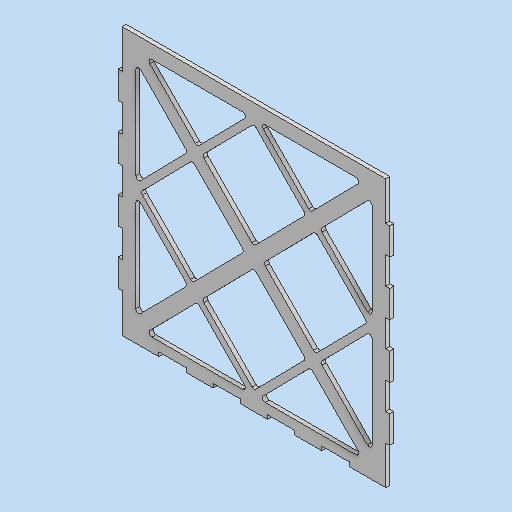
# Autodesk Inventor part: left plate
Saved by Autodesk Inventor 2026 (Build 300175000, 175)
## iProperties
Created: 2026-02-12
Part Number: left plate
Material: Generic
Document SubType Name: Modeling
Designer: mones
Density: 1 g/cm^3
Appearance: Default
Author: mones
Autodesk Inventor part; units mm, degrees
ref_plane "YZ Plane" through (0, 0, 0) normal (1, 0, 0) x (0, 1, 0)
ref_plane "XZ Plane" through (0, 0, 0) normal (0, 1, 0) x (-1, 0, 0)
ref_plane "XY Plane" through (0, 0, 0) normal (0, 0, 1) x (1, 0, 0)
sketch "Sketch1" plane through (0, 0, 0) normal (0, 0, 1) x (1, 0, 0)
  line L0 (-97, 98.5) -> (97, 98.5)
  line L1 (-100, 98.5) -> (100, -98.5) construction
  line L2 (100, 98.5) -> (-100, -98.5) construction
  line L3 (-97, 98.5) -> (-97, 70)
  line L4 (-97, 50) -> (-97, 30)
  line L5 (-97, 10) -> (-97, -10)
  line L6 (-97, -70) -> (-97, -98.5)
  line L7 (-97, 70) -> (-100, 70)
  line L8 (-100, 70) -> (-100, 50)
  line L9 (-100, 30) -> (-100, 10)
  line L10 (-100, -10) -> (-100, -30)
  line L11 (-100, -50) -> (-100, -70)
  line L12 (-100, -70) -> (-97, -70)
  line L13 (-100, -50) -> (-97, -50)
  line L14 (-100, -30) -> (-97, -30)
  line L15 (-100, -10) -> (-97, -10)
  line L16 (-100, 10) -> (-97, 10)
  line L17 (-100, 30) -> (-97, 30)
  line L18 (-100, 50) -> (-97, 50)
  line L19 (97, 98.5) -> (97, 70)
  line L20 (97, 50) -> (97, 30)
  line L21 (97, 10) -> (97, -10)
  line L22 (97, -30) -> (97, -50)
  line L23 (97, -70) -> (97, -98.5)
  line L24 (97, 70) -> (100, 70)
  line L25 (100, 70) -> (100, 50)
  line L26 (100, 30) -> (100, 10)
  line L27 (100, -10) -> (100, -30)
  line L28 (100, -50) -> (100, -70)
  line L29 (100, -70) -> (97, -70)
  line L30 (100, -50) -> (97, -50)
  line L31 (100, -30) -> (97, -30)
  line L32 (100, -10) -> (97, -10)
  line L33 (100, 10) -> (97, 10)
  line L34 (100, 30) -> (97, 30)
  line L35 (100, 50) -> (97, 50)
  line L36 (-100, 50) -> (-100, 70)
  line L37 (-97, 98.5) -> (-97, 70)
  line L38 (-97, 50) -> (-97, 30)
  line L39 (-100, 10) -> (-100, 30)
  line L40 (-97, 10) -> (-97, -10)
  line L41 (-100, -70) -> (-100, -50)
  line L42 (-100, -30) -> (-100, -10)
  line L43 (-97, -30) -> (-97, -50)
  line L44 (-97, -70) -> (-97, -98.5)
  line L45 (100, 50) -> (100, 70)
  line L46 (100, 70) -> (100, 50)
  line L47 (97, 98.5) -> (97, 70)
  line L48 (97, 50) -> (97, 30)
  line L49 (100, 30) -> (100, 10)
  line L50 (100, 10) -> (100, 30)
  line L51 (97, 10) -> (97, -10)
  line L52 (100, -70) -> (100, -50)
  line L53 (100, -30) -> (100, -10)
  line L54 (100, -10) -> (100, -30)
  line L55 (100, -50) -> (100, -70)
  line L56 (97, -30) -> (97, -50)
  line L57 (97, -70) -> (97, -98.5)
  line L58 (-97, -98.5) -> (-70, -98.5)
  line L59 (-50, -98.5) -> (-30, -98.5)
  line L60 (-10, -98.5) -> (10, -98.5)
  line L61 (30, -98.5) -> (50, -98.5)
  line L62 (-97, -98.5) -> (-97, -95.5)
  line L63 (-97, -95.5) -> (97, -95.5) construction
  line L64 (-70, -98.5) -> (-70, -95.5)
  line L65 (-50, -98.5) -> (-50, -95.5)
  line L66 (-30, -98.5) -> (-30, -95.5)
  line L67 (-10, -98.5) -> (-10, -95.5)
  line L68 (10, -98.5) -> (10, -95.5)
  line L69 (30, -98.5) -> (30, -95.5)
  line L70 (50, -98.5) -> (50, -95.5)
  line L71 (70, -98.5) -> (70, -95.5)
  line L72 (97, -98.5) -> (70, -98.5)
  line L73 (50, -95.5) -> (70, -95.5)
  line L74 (50, -98.5) -> (30, -98.5)
  line L75 (10, -95.5) -> (30, -95.5)
  line L76 (10, -98.5) -> (-10, -98.5)
  line L77 (-70, -95.5) -> (-50, -95.5)
  line L78 (-30, -95.5) -> (-10, -95.5)
  line L79 (-30, -98.5) -> (-50, -98.5)
  line L80 (-70, -98.5) -> (-97, -98.5)
  point P0 (0, 0)
  constraints: 160 end point, 58 perpendicular, 28 parallel, 2 midpoint, 2 vertical, 1 horizontal, 1 point on line, 11 other
extrude "Extrusion1" add sketch "Sketch1" along normal blind 3
sketch "Sketch2" plane through (0, 0, 3) normal (0, 0, 1) x (1, 0, 0)
  line L0 (-97, 98.5) -> (-97, 70) projected
  line L1 (-97, 70) -> (-100, 70) projected
  line L2 (-100, 70) -> (-100, 50) projected
  line L3 (-100, 50) -> (-97, 50) projected
  line L4 (-97, 50) -> (-97, 30) projected
  line L5 (-97, 30) -> (-100, 30) projected
  line L6 (-100, 30) -> (-100, 10) projected
  line L7 (-100, 10) -> (-97, 10) projected
  line L8 (-97, 10) -> (-97, -10) projected
  line L9 (-97, -10) -> (-100, -10) projected
  line L10 (-100, -10) -> (-100, -30) projected
  line L11 (-100, -30) -> (-97, -30) projected
  line L12 (-97, -30) -> (-97, -50) projected
  line L13 (-97, -50) -> (-100, -50) projected
  line L14 (-100, -50) -> (-100, -70) projected
  line L15 (-100, -70) -> (-97, -70) projected
  line L16 (-97, -70) -> (-97, -98.5) projected
  line L17 (-97, -98.5) -> (-70, -98.5) projected
  line L18 (-70, -98.5) -> (-70, -95.5) projected
  line L19 (-70, -95.5) -> (-50, -95.5) projected
  line L20 (-50, -95.5) -> (-50, -98.5) projected
  line L21 (-50, -98.5) -> (-30, -98.5) projected
  line L22 (-30, -98.5) -> (-30, -95.5) projected
  line L23 (-30, -95.5) -> (-10, -95.5) projected
  line L24 (-10, -95.5) -> (-10, -98.5) projected
  line L25 (-10, -98.5) -> (10, -98.5) projected
  line L26 (10, -98.5) -> (10, -95.5) projected
  line L27 (10, -95.5) -> (30, -95.5) projected
  line L28 (30, -95.5) -> (30, -98.5) projected
  line L29 (30, -98.5) -> (50, -98.5) projected
  line L30 (50, -98.5) -> (50, -95.5) projected
  line L31 (50, -95.5) -> (70, -95.5) projected
  line L32 (70, -95.5) -> (70, -98.5) projected
  line L33 (70, -98.5) -> (97, -98.5) projected
  line L34 (97, -98.5) -> (97, -70) projected
  line L35 (97, -70) -> (100, -70) projected
  line L36 (100, -70) -> (100, -50) projected
  line L37 (100, -50) -> (97, -50) projected
  line L38 (97, -50) -> (97, -30) projected
  line L39 (97, -30) -> (100, -30) projected
  line L40 (100, -30) -> (100, -10) projected
  line L41 (100, -10) -> (97, -10) projected
  line L42 (97, -10) -> (97, 10) projected
  line L43 (97, 10) -> (100, 10) projected
  line L44 (100, 10) -> (100, 30) projected
  line L45 (100, 30) -> (97, 30) projected
  line L46 (97, 30) -> (97, 50) projected
  line L47 (97, 50) -> (100, 50) projected
  line L48 (100, 50) -> (100, 70) projected
  line L49 (100, 70) -> (97, 70) projected
  line L50 (97, 70) -> (97, 98.5) projected
  line L51 (97, 98.5) -> (-97, 98.5) projected
  line L52 (-97, 98.5) -> (97, 98.5)
  line L53 (97, 98.5) -> (97, -98.5)
  line L54 (97, -98.5) -> (-97, -98.5)
  line L55 (-97, -98.5) -> (-97, 98.5)
  line L56 (-90.5656, -84.9948) -> (90.5656, 84.9948) construction
  line L57 (-90.5656, 84.9948) -> (90.5656, -84.9948) construction
  line L58 (83.4344, -92.0052) -> (-83.4344, 92.0052) construction
  line L59 (1.7528, 86.7169) -> (1.7516, 86.7182)
  line L60 (-88.7828, -1.7526) -> (0, -85.0743) construction
  line L61 (-1.7828, -90.2526) -> (-85.2172, 1.7526) construction
  line L62 (85.2172, 1.7526) -> (1.7828, -90.2526) construction
  line L63 (85.2172, -1.7526) -> (1.7828, 90.2526) construction
  line L64 (-88.7828, 1.7526) -> (1.7828, 86.7474) construction
  line L65 (-1.7828, 90.2526) -> (-85.2172, -1.7526) construction
  line L66 (75.2179, 88.5) -> (8.2764, 88.5)
  line L67 (-8.2764, 88.5) -> (-75.2179, 88.5)
  line L68 (87, -76.4803) -> (87, -8.4535)
  line L69 (87, 8.4535) -> (87, 76.4803)
  line L70 (6.8501, -85.0979) -> (40.3209, -51.0501)
  line L71 (50.1369, -41.0649) -> (83.5738, -7.0515)
  line L72 (82.116, -1.4021) -> (46.6791, -37.4499)
  line L73 (43.1734, -51.0501) -> (76.6442, -85.0979)
  line L74 (40.3209, 51.0501) -> (6.8501, 85.0979)
  line L75 (46.6791, 37.4499) -> (82.116, 1.4021)
  line L76 (83.5738, 7.0515) -> (50.1369, 41.0649)
  line L77 (83.5738, 77.8824) -> (50.1369, 43.869)
  line L78 (83.4344, 92.0052) -> (41.6783, 45.9597) construction
  line L79 (3.3643, 3.7099) -> (-83.4344, -92.0052) construction
  line L80 (43.1734, 51.0501) -> (76.6442, 85.0979)
  line L81 (1.4262, 83.483) -> (36.8631, 47.4351)
  line L82 (-1.7828, 86.7474) -> (-1.7516, 86.7182) construction
  line L83 (0, 85.0743) -> (88.7828, 1.7526) construction
  line L84 (-1.4262, 83.483) -> (-36.8631, 47.4351)
  line L85 (-46.6791, 37.4499) -> (-82.116, 1.4021)
  line L86 (-43.1734, 51.0501) -> (-76.6442, 85.0979)
  line L87 (-83.5738, 7.0515) -> (-50.1369, 41.0649)
  line L88 (-40.3209, 51.0501) -> (-6.8501, 85.0979)
  line L89 (-83.5738, 77.8824) -> (-50.1369, 43.869)
  line L90 (-87, 76.4803) -> (-87, 8.4535)
  line L91 (-87, -8.4535) -> (-87, -76.4803)
  line L92 (36.8631, -47.4351) -> (1.4262, -83.483)
  line L93 (-75.2179, -88.5) -> (-8.2764, -88.5)
  line L94 (8.2764, -88.5) -> (75.2179, -88.5)
  line L95 (0, -85.0743) -> (88.7828, -1.7526) construction
  line L96 (-83.5738, -7.0515) -> (-50.1369, -41.0649)
  line L97 (-40.3209, -51.0501) -> (-6.8501, -85.0979)
  line L98 (-1.4262, -83.483) -> (-36.8631, -47.4351)
  line L99 (-46.6791, -37.4499) -> (-82.116, -1.4021)
  line L100 (-43.1734, -51.0501) -> (-76.6442, -85.0979)
  line L101 (-83.5738, -77.8824) -> (-50.1369, -43.869)
  line L102 (43.8266, 37.4499) -> (8.3897, 1.4021)
  line L103 (-1.4262, 8.5831) -> (-36.8631, 44.631)
  line L104 (-1.4262, -8.5831) -> (-36.8631, -44.631)
  line L105 (-43.8266, 37.4499) -> (-8.3897, 1.4021)
  line L106 (1.4262, -8.5831) -> (36.8631, -44.631)
  line L107 (-43.8266, -37.4499) -> (-8.3897, -1.4021)
  line L108 (1.4262, 8.5831) -> (36.8631, 44.631)
  line L109 (83.5738, -77.8824) -> (50.1369, -43.869)
  line L110 (43.8266, -37.4499) -> (8.3897, -1.4021)
  arc A0 (-83.5738, 77.8824) -> (-87, 76.4803) centre (-85, 76.4803) ccw
  arc A1 (-50.1369, 41.0649) -> (-50.1369, 43.869) centre (-51.5631, 42.4669) ccw
  arc A2 (-87, 8.4535) -> (-83.5738, 7.0515) centre (-85, 8.4535) ccw
  arc A3 (-43.8266, 37.4499) -> (-46.6791, 37.4499) centre (-45.2528, 36.0479) ccw
  arc A4 (-82.116, 1.4021) -> (-82.116, -1.4021) centre (-80.6897, 0) ccw
  arc A5 (-8.3897, -1.4021) -> (-8.3897, 1.4021) centre (-9.816, 0) ccw
  arc A6 (-46.6791, -37.4499) -> (-43.8266, -37.4499) centre (-45.2528, -36.0479) ccw
  arc A7 (-83.5738, -7.0515) -> (-87, -8.4535) centre (-85, -8.4535) ccw
  arc A8 (-50.1369, -43.869) -> (-50.1369, -41.0649) centre (-51.5631, -42.4669) ccw
  arc A9 (-87, -76.4803) -> (-83.5738, -77.8824) centre (-85, -76.4803) ccw
  arc A10 (-40.3209, -51.0501) -> (-43.1734, -51.0501) centre (-41.7472, -52.4521) ccw
  arc A11 (-8.2764, -88.5) -> (-6.8501, -85.0979) centre (-8.2764, -86.5) ccw
  arc A12 (-76.6442, -85.0979) -> (-75.2179, -88.5) centre (-75.2179, -86.5) ccw
  arc A13 (6.8501, -85.0979) -> (8.2764, -88.5) centre (8.2764, -86.5) ccw
  arc A14 (75.2179, -88.5) -> (76.6442, -85.0979) centre (75.2179, -86.5) ccw
  arc A15 (43.1734, -51.0501) -> (40.3209, -51.0501) centre (41.7472, -52.4521) ccw
  arc A16 (36.8631, -47.4351) -> (36.8631, -44.631) centre (35.4369, -46.0331) ccw
  arc A17 (1.4262, -8.5831) -> (-1.4262, -8.5831) centre (0, -9.9852) ccw
  arc A18 (-36.8631, -44.631) -> (-36.8631, -47.4351) centre (-35.4369, -46.0331) ccw
  arc A19 (-1.4262, -83.483) -> (1.4262, -83.483) centre (0, -82.0809) ccw
  arc A20 (8.3897, 1.4021) -> (8.3897, -1.4021) centre (9.816, 0) ccw
  arc A21 (46.6791, 37.4499) -> (43.8266, 37.4499) centre (45.2528, 36.0479) ccw
  arc A22 (82.116, -1.4021) -> (82.116, 1.4021) centre (80.6897, 0) ccw
  arc A23 (43.8266, -37.4499) -> (46.6791, -37.4499) centre (45.2528, -36.0479) ccw
  arc A24 (50.1369, -41.0649) -> (50.1369, -43.869) centre (51.5631, -42.4669) ccw
  arc A25 (83.5738, -77.8824) -> (87, -76.4803) centre (85, -76.4803) ccw
  arc A26 (87, -8.4535) -> (83.5738, -7.0515) centre (85, -8.4535) ccw
  arc A27 (83.5738, 7.0515) -> (87, 8.4535) centre (85, 8.4535) ccw
  arc A28 (87, 76.4803) -> (83.5738, 77.8824) centre (85, 76.4803) ccw
  arc A29 (50.1369, 43.869) -> (50.1369, 41.0649) centre (51.5631, 42.4669) ccw
  arc A30 (76.6442, 85.0979) -> (75.2179, 88.5) centre (75.2179, 86.5) ccw
  arc A31 (8.2764, 88.5) -> (6.8501, 85.0979) centre (8.2764, 86.5) ccw
  arc A32 (40.3209, 51.0501) -> (43.1734, 51.0501) centre (41.7472, 52.4521) ccw
  arc A33 (36.8631, 44.631) -> (36.8631, 47.4351) centre (35.4369, 46.0331) ccw
  arc A34 (-1.4262, 8.5831) -> (1.4262, 8.5831) centre (0, 9.9852) ccw
  arc A35 (-36.8631, 47.4351) -> (-36.8631, 44.631) centre (-35.4369, 46.0331) ccw
  arc A36 (1.4262, 83.483) -> (-1.4262, 83.483) centre (0, 82.0809) ccw
  arc A37 (-6.8501, 85.0979) -> (-8.2764, 88.5) centre (-8.2764, 86.5) ccw
  arc A38 (-75.2179, 88.5) -> (-76.6442, 85.0979) centre (-75.2179, 86.5) ccw
  arc A39 (-43.1734, 51.0501) -> (-40.3209, 51.0501) centre (-41.7472, 52.4521) ccw
  point P0 (87, -81.6485)
  point P1 (80.2557, -88.5)
  point P2 (0.0718, 85.0069)
  point P3 (-0.0718, 85.0069)
  dimension "d39" = 2
  constraints: 118 end point, 80 point on circle, 80 tangent, 58 parallel, 40 centre point, 39 equal radius, 11 point on line, 5 perpendicular, 1 horizontal
  measures "d39" radius of A0
extrude "Extrusion2" cut sketch "Sketch2" against normal blind 3 contours A30 L80 A32 L74 A31 L66 | A37 L88 A39 L86 A38 L67 | A25 L109 A24 L71 A26 L68 | A27 L76 A29 L77 A28 L69 | L70 A15 L73 A14 L94 A13 | L72 A23 L110 A20 L102 A21 L75 A22 | L81 A33 L108 A34 L103 A35 L84 A36 | A3 L105 A5 L107 A6 L99 A4 L85 | A2 L90 A0 L89 A1 L87 | A7 L96 A8 L101 A9 L91 | L92 A19 L98 A18 L104 A17 L106 A16 | A12 L100 A10 L97 A11 L93
body "Solid1"
